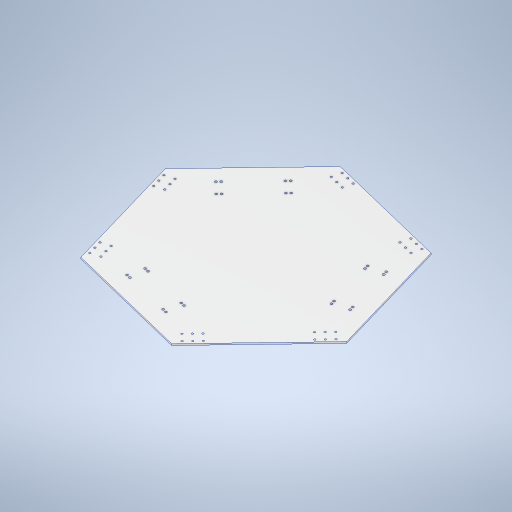
# Autodesk Inventor part: ArmPlatform
Saved by Autodesk Inventor 2024 (Build 280153000, 153)
## iProperties
Created: 2023-11-19
Part Number: ArmPlatform
Material: Aluminum 6061
Document SubType Name: Modeling
Designer: pratikhya
Density: 2.7 g/cm^3
Appearance: Aluminum - Flat
Mass: 980.019 g
Surface Area: 1502.04 cm^2
Volume: 362.97 cm^3
Sending System: SolidWorks 2021
Last Author: mrl-iitk
Last Saved: 2023-12-06
Author: pratikhya
Autodesk Inventor part; units mm, degrees
ref_plane "YZ Plane" through (0, 0, 0) normal (1, 0, 0) x (0, 1, 0)
ref_plane "XZ Plane" through (0, 0, 0) normal (0, 1, 0) x (-1, 0, 0)
ref_plane "XY Plane" through (0, 0, 0) normal (0, 0, 1) x (1, 0, 0)
ref_plane "Work Plane2" through (-4.4547, 5, 22.3935) normal (0, 1, 0) x (0.9711, 0, 0.2385)
sketch "Sketch2" plane through (-4.4547, 5, 22.3935) normal (0, 1, 0) x (0.9711, 0, 0.2385)
  line L0 (1.3055, 292.2458) -> (0.897, 292.9749)
  line L1 (165, 0) -> (82.5, 142.8942)
  line L2 (165, 0) -> (455.412, 0) construction
  line L3 (-165, 0) -> (-123.75, 71.4471)
  line L4 (-82.5, 142.8942) -> (82.5, 142.8942)
  line L5 (165, 0) -> (82.5384, -142.8363)
  line L6 (-165, 0) -> (-82.4975, -142.8985)
  line L7 (-82.4975, -142.8985) -> (82.5384, -142.8363)
  line L8 (-123.75, 71.4471) -> (123.7519, -71.4482)
  line L9 (-123.75, 71.4471) -> (-82.5, 142.8942)
  line L10 (-123.75, 71.4471) -> (-103.596, 106.3548)
  line L11 (-103.596, 106.3548) -> (-143.904, 36.5393)
  line L12 (-143.904, 36.5393) -> (-20.154, -34.9078)
  line L13 (-143.904, 36.5393) -> (-141.404, 40.8695)
  line L14 (-141.404, 40.8695) -> (-13.7235, -32.8469)
  line L15 (-143.904, 36.5393) -> (-140.154, 43.0345)
  line L16 (-140.154, 43.0345) -> (-8.7235, -32.8469)
  circle A0 centre (-122.1364, 29.7453) radius 1.25
  line L17 (-122.1364, 29.7453) -> (-104.8159, 19.7453)
  circle A1 centre (-104.8159, 19.7453) radius 1.25
  circle A2 centre (-119.6364, 34.0755) radius 1.25
  circle A3 centre (-102.3159, 24.0755) radius 1.25
  circle A4 centre (-86.8284, 90.9006) radius 1.25
  circle A5 centre (-69.5079, 80.9006) radius 1.25
  circle A6 centre (-72.0079, 76.5705) radius 1.25
  circle A7 centre (-89.3284, 86.5705) radius 1.25
  line L18 (-103.596, 106.3548) -> (38.9161, 24.0755)
  line L19 (0, -168.5342) -> (0, 201.2918)
  circle A8 centre (122.1364, 29.7453) radius 1.25
  circle A9 centre (104.8159, 19.7453) radius 1.25
  circle A10 centre (102.3159, 24.0755) radius 1.25
  circle A11 centre (119.6364, 34.0755) radius 1.25
  circle A12 centre (72.0079, 76.5705) radius 1.25
  circle A13 centre (89.3284, 86.5705) radius 1.25
  circle A14 centre (86.8284, 90.9006) radius 1.25
  circle A15 centre (69.5079, 80.9006) radius 1.25
  circle A16 centre (-35.308, -100.6459) radius 1.25
  circle A17 centre (30.308, -100.6459) radius 1.25
  circle A18 centre (35.308, -100.6459) radius 1.25
  circle A19 centre (30.308, -120.6459) radius 1.25
  circle A20 centre (35.308, -120.6459) radius 1.25
  circle A21 centre (-30.308, -100.6459) radius 1.25
  circle A22 centre (-30.308, -120.6459) radius 1.25
  circle A23 centre (-35.308, -120.6459) radius 1.25
  line L20 (-82.4975, -142.8985) -> (-65.177, -132.8985)
  line L21 (-82.4975, -142.8985) -> (-79.0334, -140.8985)
  line L22 (-165, 0) -> (-147.6795, 10)
  line L23 (-165, 0) -> (-145, 0) construction
  line L24 (-147.6795, 10) -> (-65.177, -132.8985)
  line L25 (-165, 0) -> (-161.5359, 2)
  line L26 (-161.5359, 2) -> (-79.0334, -140.8985)
  line L27 (-73.8372, -137.8985) -> (-156.3397, 5)
  line L28 (-79.0334, -140.8985) -> (-84.0334, -132.2383)
  line L29 (-84.0334, -132.2383) -> (-89.0334, -123.578)
  line L30 (-89.0334, -123.578) -> (-94.0334, -114.9178)
  line L31 (-123.7487, -71.4493) -> (-106.4282, -61.4493)
  circle A24 centre (-84.0334, -132.2383) radius 1.25
  circle A25 centre (-89.0334, -123.578) radius 1.25
  circle A26 centre (-94.0334, -114.9178) radius 1.25
  circle A27 centre (-73.6411, -126.2383) radius 1.25
  circle A28 centre (-78.6411, -117.578) radius 1.25
  circle A29 centre (-83.6411, -108.9178) radius 1.25
  circle A30 centre (-156.5359, -6.6603) radius 1.25
  circle A31 centre (-151.5359, -15.3205) radius 1.25
  circle A32 centre (-146.5359, -23.9808) radius 1.25
  circle A33 centre (-136.1436, -17.9808) radius 1.25
  circle A34 centre (-141.1436, -9.3205) radius 1.25
  circle A35 centre (-146.1436, -0.6603) radius 1.25
  circle A36 centre (72.505, 138.8942) radius 1.25
  circle A37 centre (62.505, 138.8942) radius 1.25
  circle A38 centre (52.505, 138.8942) radius 1.25
  circle A39 centre (52.505, 126.8942) radius 1.25
  circle A40 centre (62.505, 126.8942) radius 1.25
  circle A41 centre (72.505, 126.8942) radius 1.25
  circle A42 centre (-72.5, 138.8942) radius 1.25
  circle A43 centre (-62.5, 138.8942) radius 1.25
  circle A44 centre (-52.5, 138.8942) radius 1.25
  circle A45 centre (-52.5, 126.8942) radius 1.25
  circle A46 centre (-62.5, 126.8942) radius 1.25
  circle A47 centre (-72.5, 126.8942) radius 1.25
  circle A48 centre (84.0334, -132.2383) radius 1.25
  circle A49 centre (89.0334, -123.578) radius 1.25
  circle A50 centre (94.0334, -114.9178) radius 1.25
  circle A51 centre (83.6411, -108.9178) radius 1.25
  circle A52 centre (78.6411, -117.578) radius 1.25
  circle A53 centre (73.6411, -126.2383) radius 1.25
  circle A54 centre (156.5359, -6.6603) radius 1.25
  circle A55 centre (151.5359, -15.3205) radius 1.25
  circle A56 centre (146.5359, -23.9808) radius 1.25
  circle A57 centre (136.1436, -17.9808) radius 1.25
  circle A58 centre (141.1436, -9.3205) radius 1.25
  circle A59 centre (146.1436, -0.6603) radius 1.25
  dimension "d14" = 120
  dimension "d19" = 40.308
  dimension "d20" = 80.616
  dimension "d21" = 5
  dimension "d22" = 7.5
  dimension "d23" = 2.5
  dimension "d24" = 20
  dimension "d25" = 2.5
  dimension "d40" = 20
  dimension "d42" = 4
  dimension "d43" = 90
  dimension "d45" = 20
  dimension "d46" = 30
  dimension "d47" = 10
  dimension "d48" = 10
  dimension "d50" = 10
  dimension "d51" = 2.5
  dimension "d52" = 2.5
  dimension "d53" = 2.5
  constraints: 64 end point, 60 centre point, 55 symmetric about line, 12 point on line, 4 coincident, 4 midpoint, 4 perpendicular, 3 horizontal, 1 equal length, 1 parallel, 1 vertical, 55 other
  measures "d14" angle of L2 L1
  measures "d19" distance of L3.end L10.end
  measures "d20" distance of L10.end L11.end
  measures "d21" distance of L11.end L13.end
  measures "d22" distance of L11.end L15.end
  measures "d23" diameter of A0
  measures "d24" distance of L17.start L17.end
  measures "d25" diameter of A1
  measures "d40" distance of L6.end L20.end
  measures "d42" distance of L6.end L21.end
  measures "d43" angle of L6 L20
  measures "d45" distance of L3.start L22.end
  measures "d46" angle of L23 L22
  measures "d47" distance of L21.end L28.end
  measures "d48" distance of L28.end L29.end
  measures "d50" distance of L29.end L30.end
  measures "d51" diameter of A24
  measures "d52" diameter of A25
  measures "d53" diameter of A26
ref_plane "Work Plane3" through (-4.4547, 5, 22.3935) normal (0, 1, 0) x (0.9711, 0, 0.2385)
extrude "Extrusion2" add sketch "Sketch2" along normal blind 2 contours L5 L8 L19 L4 L1 | L5 L7 L19 L8 | L19 L18 L9 L4 | A1 L14 | L14 A1 | A0 L14 | L14 A0 | L19 L7 L20 L24 L22 L3 L8 | L8 L9 L18 L19 | L6 L31 L26 A26 A25 A24 L20 | L6 L22 L26 A30 A31 A32 L31 | L26 A24 A25 A26 L31 L27 L20 | L26 A32 A31 A30 L22 L27 L31 | L27 L31 L24 L20 | A24 L26 | L26 A24 | A32 L26 | L26 A32 | A26 L26 | L26 A26 | L27 L22 L24 L31 | A30 L26 | L26 A30 | A25 L26 | L26 A25 | A31 L26 | L26 A31 | A2 | A3 | A4 | A5 | A6 | A7 | A8 | A9 | A10 | A11 | A12 | A13 | A14 | A15 | A16 | A17 | A18 | A19 | A20 | A21 | A22 | A23 | A27 | A28 | A29 | A33 | A34 | A35 | A36 | A37 | A38 | A39 | A40 | A41 | A42 | A43 | A44 | A45 | A46 | A47 | A48 | A49 | A50 | A51 | A52 | A53 | A54 | A55 | A56 | A57 | A58 | A59
hole "Hole1" at (-98.0768, 5, -25.3881) at (-112.5127, 5, -39.2302) at (-115.9733, 5, -35.6213) at (-101.5374, 5, -21.7791) at (-70.56, 5, -82.9826) at (-67.0994, 5, -86.5915) at (-52.6635, 5, -72.7494) at (-56.1241, 5, -69.1404) direction (0, 1, 0) diameter 3 end through all
hole "Hole2" at (-67.5161, 5, 131.1379) at (-62.6604, 5, 132.3303) at (-62.7464, 5, 111.715) at (-57.8907, 5, 112.9074) at (-3.7934, 5, 146.7863) at (1.0623, 5, 147.9787) at (5.832, 5, 128.5558) at (0.9763, 5, 127.3634) at (102.0458, 5, 28.2148) at (100.6506, 5, 23.4134) at (121.2514, 5, 22.634) at (119.8562, 5, 17.8326) at (83.7364, 5, -34.7949) at (82.3412, 5, -39.5963) at (102.942, 5, -40.3757) at (101.5468, 5, -45.1771) direction (0, 1, 0) diameter 3 end through all
hole "Hole3" at (-44.6005, 5, -118.1295) at (-34.8891, 5, -115.7446) at (-25.1776, 5, -113.3598) at (-22.3158, 5, -125.0136) at (-32.0273, 5, -127.3984) at (-41.7387, 5, -129.7832) at (79.6595, 5, -99.9715) at (76.7976, 5, -88.3177) at (86.5091, 5, -85.9329) at (89.3709, 5, -97.5866) at (99.0824, 5, -95.2018) at (96.2206, 5, -83.548) at (-152.4816, 5, 10.7358) at (-140.9582, 5, 7.3873) at (-143.7486, 5, -2.2155) at (-155.2719, 5, 1.133) at (-158.0623, 5, -8.4698) at (-146.539, 5, -11.8183) at (-123.181, 5, 111.5699) at (-111.6576, 5, 108.2215) at (-108.8672, 5, 117.8243) at (-106.0769, 5, 127.4271) at (-117.6002, 5, 130.7755) at (-120.3906, 5, 121.1727) at (36.9557, 5, 162.5516) at (45.6172, 5, 170.8568) at (52.5383, 5, 163.6389) at (43.8767, 5, 155.3336) at (50.7978, 5, 148.1157) at (59.4593, 5, 156.4209) at (132.134, 5, 80.6288) at (123.4725, 5, 72.3235) at (130.3936, 5, 65.1056) at (139.0551, 5, 73.4109) at (145.9762, 5, 66.1929) at (137.3146, 5, 57.8876) direction (0, 1, 0) diameter 2.5 end through all
body "Solid3"
